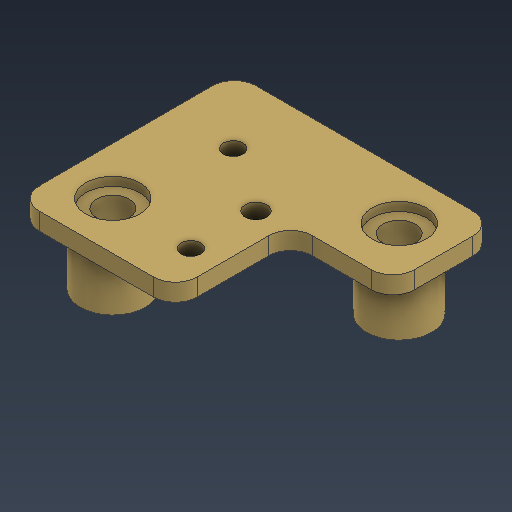
# Autodesk Inventor part: Chapa Intermediária
Saved by Autodesk Inventor 2021 (Build 250183000, 183)
## iProperties
Created: 2021-01-18
Part Number: Chapa Intermediária
Material: Genérico
Document SubType Name: Modeling
Designer: João
Density: 1 g/cm^3
Appearance: Padrão
Author: João
Autodesk Inventor part; units mm, degrees
ref_plane "YZ Plane" through (0, 0, 0) normal (1, 0, 0) x (0, 1, 0)
ref_plane "XZ Plane" through (0, 0, 0) normal (0, 1, 0) x (-1, 0, 0)
ref_plane "XY Plane" through (0, 0, 0) normal (0, 0, 1) x (1, 0, 0)
sketch "Esboço1" plane through (0, 0, 0) normal (0, 1, 0) x (-1, 0, 0)
  arc A0 (-0.2821, 5) -> (-1.282, 4) centre (-0.282, 4) ccw
  line L0 (-1.282, 4) -> (-1.282, 0.6875)
  arc A1 (-2.282, -0.3125) -> (-1.282, 0.6875) centre (-2.282, 0.6875) ccw
  line L1 (-2.282, -0.3125) -> (-5, -0.3125)
  arc A2 (-5, -0.3125) -> (-6, -1.3125) centre (-5, -1.3125) ccw
  line L2 (-6, -1.3125) -> (-6, -4)
  arc A3 (-6, -4) -> (-5, -5) centre (-5, -4) ccw
  line L3 (-5, -5) -> (5, -5)
  arc A4 (5, -5) -> (6, -4) centre (5, -4) ccw
  line L4 (6, -4) -> (6, 4)
  arc A5 (6, 4) -> (5, 5) centre (5, 4) ccw
  line L5 (5, 5) -> (-0.2821, 5)
  circle A6 centre (3.0146, -1.9633) radius 0.45
  circle A7 centre (-3.8014, -2.7994) radius 1.25
  circle A8 centre (3.8014, 2.7994) radius 1.25
  circle A9 centre (3.8014, 2.7994) radius 1.25
  circle A10 centre (3.8014, 2.7994) radius 0.75
  circle A11 centre (-3.8014, -2.7994) radius 1.25
  circle A12 centre (-3.8014, -2.7994) radius 0.75
  circle A13 centre (0, 0) radius 0.5
  circle A14 centre (0, 3) radius 0.45
  dimension "d9" = 1
  dimension "d12" = 0.9
  dimension "d13" = 2
  constraints: 15 centre point, 12 end point, 12 point on circle
  measures "d9" diameter of A13
  measures "d12" diameter of A14
  measures "d13" distance from line of L5 A14.centre
extrude "Extrusão1" add sketch "Esboço1" along normal blind 0.8 contours L5 A5 L4 A4 L3 A3 L2 A2 L1 A1 L0 A0 | A14
extrude "Extrusão2" add sketch "Esboço1" along normal blind 0.4 contours A7 | A8
sketch "Esboço2" plane through (0, 0, 0) normal (0, -1, 0) x (1, 0, 0)
  circle A0 centre (-3.8014, 2.7994) radius 0.75 projected
  circle A1 centre (-3.8014, 2.7994) radius 1.5
  circle A2 centre (3.8014, -2.7994) radius 0.75 projected
  circle A3 centre (3.8014, -2.7994) radius 1.5
  point P0 (0, 0)
  dimension "d4" = 3
  dimension "d5" = 3
  constraints: 2 centre point, 2 coincident
  measures "d4" diameter of A1
  measures "d5" diameter of A3
extrude "Extrusão3" add sketch "Esboço2" along normal blind 2.8
extrude "Extrusão4" cut sketch "Esboço1" along normal blind 10 contours A14
